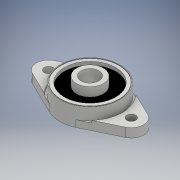
# Autodesk Inventor part: KFL08
Saved by Autodesk Inventor 2018 (Build 220112000, 112)
## iProperties
Created: 2018-09-20
Part Number: KFL08
Material: Genérico
Document SubType Name: Modeling
Designer: Georgines
Density: 1 g/cm^3
Appearance: Padrão
Author: Georgines
Autodesk Inventor part; units mm, degrees
ref_plane "YZ Plane" through (0, 0, 0) normal (1, 0, 0) x (0, 1, 0)
ref_plane "XZ Plane" through (0, 0, 0) normal (0, 1, 0) x (-1, 0, 0)
ref_plane "XY Plane" through (0, 0, 0) normal (0, 0, 1) x (1, 0, 0)
sketch "Esboço1" plane through (0, 0, 0) normal (0, 0, 1) x (1, 0, 0)
  line L0 (-18.5, 0) -> (18.5, 0) construction
  line L1 (-24, 0) -> (24, 0) construction
  line L2 (-20.8784, 4.9592) -> (-5.7013, 12.238)
  line L3 (20.8784, 4.9592) -> (5.8378, 12.1725)
  line L4 (-20.8784, -4.9592) -> (-5.5742, -12.299)
  line L5 (5.8378, -12.1725) -> (20.8784, -4.9592)
  arc A0 (20.8784, -4.9592) -> (20.8784, 4.9592) centre (18.5, 0) ccw
  arc A1 (-5.8378, -12.1725) -> (5.8378, -12.1725) centre (0, 0) ccw
  arc A2 (5.8378, 12.1725) -> (-5.8378, 12.1725) centre (0, 0) ccw
  arc A3 (-20.8784, 4.9592) -> (-20.8784, -4.9592) centre (-18.5, 0) ccw
  dimension "d1" = 37
  dimension "d2" = 48
  constraints: 12 end point, 10 point on circle, 8 tangent, 4 centre point, 4 coincident, 2 horizontal, 2 midpoint, 2 point on line
  measures "d1" distance of L0.start L0.end
  measures "d2" distance of L1.start L1.end
extrude "Extrusão1" add sketch "Esboço1" along normal blind 4
sketch "Esboço2" plane through (0, 0, 4) normal (0, 0, 1) x (1, 0, 0)
  circle A0 centre (0, 0) radius 13.5
  circle A1 centre (0, 0) radius 14.5
  dimension "d5" = 27
  dimension "d6" = 29
  constraints: 2 centre point, 2 coincident
  measures "d5" diameter of A0
  measures "d6" diameter of A1
extrude "Extrusão2" cut sketch "Esboço2" against normal blind 1
sketch "Esboço3" plane through (0, 0, 4) normal (0, 0, 1) x (1, 0, 0)
  circle A0 centre (0, 0) radius 13.5
  dimension "d9" = 27
  constraints: 1 centre point, 1 coincident
  measures "d9" diameter of A0
extrude "Extrusão3" add sketch "Esboço3" along normal blind 4.5
sketch "Esboço4" plane through (0, 0, 8.5) normal (0, 0, 1) x (1, 0, 0)
  circle A0 centre (0, 0) radius 11.5
  dimension "d12" = 23
  constraints: 1 centre point, 1 coincident
  measures "d12" diameter of A0
extrude "Extrusão4" cut sketch "Esboço4" against normal blind 1.5
sketch "Esboço5" plane through (0, 0, 0) normal (0, 0, -1) x (-1, 0, 0)
  circle A0 centre (0, 0) radius 11.5
  dimension "d15" = 23
  constraints: 1 centre point, 1 coincident
  measures "d15" diameter of A0
extrude "Extrusão5" cut sketch "Esboço5" against normal blind 1.5
sketch "Esboço6" plane through (0, 0, 8.5) normal (0, 0, 1) x (1, 0, 0)
  circle A0 centre (0, 0) radius 13
  circle A1 centre (0, 0) radius 13.25
  dimension "d18" = 26
  dimension "d19" = 26.5
  constraints: 2 centre point, 2 coincident
  measures "d18" diameter of A0
  measures "d19" diameter of A1
extrude "Extrusão6" cut sketch "Esboço6" against normal blind 0.2
sketch "Esboço8" plane through (0, 0, 0) normal (0, 0, -1) x (-1, 0, 0)
  circle A0 centre (0, 0) radius 13
  circle A1 centre (0, 0) radius 13.25
  dimension "d22" = 26
  dimension "d23" = 26.5
  constraints: 2 centre point, 2 coincident
  measures "d22" diameter of A0
  measures "d23" diameter of A1
extrude "Extrusão7" cut sketch "Esboço8" against normal blind 0.2
sketch "Esboço9" plane through (0, 0, 7) normal (0, 0, 1) x (1, 0, 0)
  circle A0 centre (0, 0) radius 6
  dimension "d26" = 12
  constraints: 1 centre point, 1 coincident
  measures "d26" diameter of A0
extrude "Extrusão8" add sketch "Esboço9" along normal blind 4
sketch "Esboço10" plane through (0, 0, 1.5) normal (0, 0, -1) x (-1, 0, 0)
  circle A0 centre (0, 0) radius 6
  dimension "d29" = 12
  constraints: 1 centre point, 1 coincident
  measures "d29" diameter of A0
extrude "Extrusão9" add sketch "Esboço10" along normal blind 1.5
sketch "Esboço11" plane through (0, 0, 11) normal (0, 0, 1) x (1, 0, 0)
  circle A0 centre (0, 0) radius 2.3758
  constraints: 1 centre point, 1 coincident
hole "Furo1" at (0, 0, 11) direction (0, 0, -1) diameter 8 end through all
sketch "Esboço12" plane through (0, 0, 0) normal (0, 0, -1) x (-1, 0, 0)
  line L0 (18.5, 0) -> (-18.5, 0) construction
  circle A0 centre (18.5, 0) radius 0.9755 construction
  circle A1 centre (-18.5, 0) radius 0.8896 construction
  point P0 (0, 0)
  point P1 (0, 0)
  dimension "d39" = 37
  constraints: 3 coincident, 2 centre point, 2 end point, 1 horizontal, 1 midpoint
  measures "d39" distance of L0.start L0.end
hole "Furo2" at (-18.5, 0, 0) at (18.5, 0, 0) direction (0, 0, 1) diameter 4 end through all
